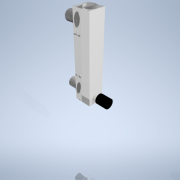
# Autodesk Inventor part: LZM-15ZT_rotameter_06-6_M3-H
Saved by Autodesk Inventor 2020 (Build 240168000, 168)
## iProperties
Created: 2020-07-28
Part Number: LZM-15ZT_rotameter_06-6_M3-H
Material: Generic
Document SubType Name: Modeling
Designer: Samuel
Density: 1 g/cm^3
Appearance: Gray
Author: Samuel
Autodesk Inventor part; units mm, degrees
ref_plane "YZ Plane" through (0, 0, 0) normal (1, 0, 0) x (0, 1, 0)
sketch "Sketch1" plane through (0, 0, 0) normal (0, 1, 0) x (-1, 0, 0)
  line L0 (-17.45, 15.95) -> (17.45, 15.95)
  line L1 (17.45, 15.95) -> (17.45, -15.95)
  line L2 (17.45, -15.95) -> (-17.45, -15.95)
  line L3 (-17.45, -15.95) -> (-17.45, 15.95)
  line L4 (-17.45, 15.95) -> (17.45, -15.95) construction
  line L5 (17.45, 15.95) -> (-17.45, -15.95) construction
  point P0 (0, 0)
  dimension "d0" = 31.9
  dimension "d1" = 34.9
  constraints: 12 end point, 2 midpoint, 2 parallel, 1 horizontal, 1 perpendicular
  measures "d0" distance of L0.end L1.end
  measures "d1" distance of L1.end L2.end
extrude "Extrusion1" add sketch "Sketch1" along normal blind 167.7
sketch "Sketch2" plane through (-17.45, 0, -15.95) normal (-1, 0, 0) x (0, 0, 1)
  line L0 (31.9, 167.7) -> (0, 167.7) projected
  line L1 (20.8388, 134.1) -> (11.0612, 157) construction
  line L2 (11.0612, 134.1) -> (20.8388, 157) construction
  arc A0 (28.2535, 143.6455) -> (8.8162, 155.7535) centre (15.95, 145.55) ccw
  arc A1 (3.6465, 147.4545) -> (23.0838, 135.3465) centre (15.95, 145.55) ccw
  line L3 (3.6465, 147.4545) -> (8.8162, 155.7535)
  line L4 (23.0838, 135.3465) -> (28.2535, 143.6455)
  point P0 (15.95, 0)
  constraints: 8 end point, 4 point on circle, 2 centre point, 2 coincident, 1 parallel
extrude "Extrusion2" add sketch "Sketch2" along normal blind 6
fillet "Fillet1" radius 0.5 8 edges at (-20.45, 147.4545, -12.3035) (-20.45, 155.7535, -7.1338) (-20.45, 143.6455, 12.3035) (-20.45, 135.3465, 7.1338) (-23.45, 134.9826, -6.5827) (-23.45, 139.496, 9.7186) (-23.45, 156.1174, 6.5827) (-23.45, 151.604, -9.7186)
sketch "Sketch4" plane through (-17.45, 0, -15.95) normal (-1, 0, 0) x (0, 0, 1)
  line L0 (31.9, 0) -> (31.9, 167.7) projected
  line L1 (31.9, 82.45) -> (0, 82.45)
  point P0 (15.95, 0)
  dimension "d13" = 85.25
  constraints: 2 end point, 1 horizontal, 1 point on line
  measures "d13" distance of L0.end L1.start
ref_plane "Work Plane2" through (-17.45, 82.45, 15.95) normal (0, 1, 0) x (0, 0, -1)
sketch "Sketch5" plane through (-23.45, 0, -15.95) normal (-1, 0, 0) x (0, 0, 1)
  line L0 (27.7744, 143.8221) -> (22.714, 135.6986) projected
  arc A0 (27.7744, 143.8221) -> (9.186, 155.4014) centre (15.95, 145.55) ccw projected
  line L1 (4.1256, 147.2779) -> (9.186, 155.4014) projected
  arc A1 (4.1256, 147.2779) -> (22.714, 135.6986) centre (15.95, 145.55) ccw projected
  circle A2 centre (15.95, 145.55) radius 10.2
  circle A3 centre (15.95, 145.55) radius 5.54
  point P0 (15.95, 0)
  dimension "d15" = 20.4
  dimension "d16" = 11.08
  constraints: 2 centre point, 1 coincident
  measures "d15" diameter of A2
  measures "d16" diameter of A3
extrude "Extrusion3" add sketch "Sketch5" along normal blind 19.7 contours A2
mirror "Mirror1" about plane through (-17.45, 82.45, 15.95) normal (0, 1, 0) of "Extrusion3", "Extrusion2", "Fillet1"
sketch "Sketch6" plane through (-17.45, 0, -15.95) normal (-1, 0, 0) x (0, 0, 1)
  circle A0 centre (15.95, 45.05) radius 4.95
  point P0 (15.95, 0)
  dimension "d21" = 9.9
  constraints: 1 centre point, 1 coincident
  measures "d21" diameter of A0
extrude "Extrusion4" cut sketch "Sketch6" against normal blind 0.7
sketch "Sketch7" plane through (-16.75, 45.05, 0) normal (-1, 0, 0) x (0, 0, 1)
  circle A0 centre (0, 0) radius 2.85
  point P0 (0, -45.05)
  dimension "d24" = 5.7
  constraints: 1 centre point
  measures "d24" diameter of A0
extrude "Extrusion5" cut sketch "Sketch7" against normal blind 7.1
sketch "Sketch8" plane through (-17.45, 0, -15.95) normal (-1, 0, 0) x (0, 0, 1)
  line L0 (0, 167.7) -> (31.9, 167.7) projected
  line L1 (0, 0) -> (0, 167.7) projected
  line L2 (0, 82.85) -> (31.9, 82.85)
  line L3 (31.9, 0) -> (31.9, 167.7) projected
  point P0 (15.95, 0)
  dimension "d27" = 84.85
  constraints: 2 end point, 2 point on line, 1 horizontal
  measures "d27" distance of L0.start L2.start
ref_plane "Work Plane3" through (-17.45, 82.85, -15.95) normal (0, -1, 0) x (0, 0, 1)
mirror "Mirror2" about plane through (-17.45, 82.85, -15.95) normal (0, -1, 0) of "Extrusion4", "Extrusion5"
thread "Thread1" size "M6x1" class "6H" standard "ANSI Metric M Profile" full length
thread "Thread2" size "M6x1" class "6H" standard "ANSI Metric M Profile" full length
thread "Thread3" size "G 1/2-14" class "A" standard "BSP Pipe Threads" full length
thread "Thread4" size "G 1/4-19" standard "BSP Pipe Threads" full length
thread "Thread5" size "G 1/2-14" class "A" standard "BSP Pipe Threads" full length
thread "Thread6" size "G 1/4-19" standard "BSP Pipe Threads" full length
sketch "Sketch9" plane through (0, 167.7, 0) normal (0, 1, 0) x (1, 0, 0)
  line L0 (17.45, -15.95) -> (17.45, 15.95) projected
  circle A0 centre (3.65, 0) radius 12.3
  point P0 (0, 0)
  dimension "d42" = 24.6
  constraints: 1 centre point, 1 coincident
  measures "d42" diameter of A0
extrude "Extrusion6" add sketch "Sketch9" along normal blind 4
fillet "Fillet2" radius 8 1 edges at (-8.65, 171.7, 0)
sketch "Sketch10" plane through (3.65, 171.7, 0) normal (0, 1, 0) x (1, 0, 0)
  line L0 (0.5, 8.73) -> (-0.5, 8.73)
  line L1 (-0.5, 8.73) -> (-0.5, -8.73)
  line L2 (-0.5, -8.73) -> (0.5, -8.73)
  line L3 (0.5, -8.73) -> (0.5, 8.73)
  circle A0 centre (0, 0) radius 5.3718 projected
  line L4 (0.5, 8.73) -> (-0.5, -8.73) construction
  line L5 (-0.5, 8.73) -> (0.5, -8.73) construction
  point P0 (-3.65, 0)
  dimension "d46" = 1
  dimension "d47" = 17.46
  constraints: 12 end point, 2 midpoint, 2 parallel, 1 horizontal, 1 perpendicular
  measures "d46" distance of L2.end L1.end
  measures "d47" distance of L1.end L0.end
extrude "Extrusion7" cut sketch "Sketch10" against normal blind 1 contours L3 A0 L1 L0 | L3 A0 L1 | L3 L2 L1 A0
sketch "Sketch11" plane through (17.45, 0, 15.95) normal (1, 0, 0) x (0, 0, -1)
  circle A0 centre (15.95, 13.63) radius 7.65
  point P0 (15.95, 0)
  dimension "d51" = 15.3
  constraints: 1 centre point, 1 coincident
  measures "d51" diameter of A0
extrude "Extrusion8" add sketch "Sketch11" along normal blind 8
sketch "Sketch12" plane through (25.45, 13.63, 0) normal (1, 0, 0) x (0, 0, -1)
  circle A0 centre (0, 0) radius 10.2
  point P0 (0, -13.63)
  dimension "d54" = 20.4
  constraints: 1 centre point
  measures "d54" diameter of A0
extrude "Extrusion9" add sketch "Sketch12" along normal blind 22.9
sketch "Sketch13" plane through (17.45, 0, 15.95) normal (1, 0, 0) x (0, 0, -1)
  line L0 (2, 162) -> (30.0498, 162) construction
  line L1 (30.0498, 162) -> (30.0498, 31.2776) construction
  line L2 (30.0498, 31.2776) -> (2, 31.2776) construction
  line L3 (2, 31.2776) -> (2, 162) construction
  point P0 (15.95, 0)
  constraints: 2 other
body "Solid1"
